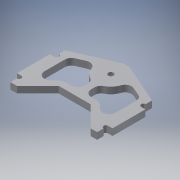
# Autodesk Inventor part: 付け根_サブフレーム_1_3
Saved by Autodesk Inventor 2018 (Build 220112000, 112)
## iProperties
Created: 2016-04-30
Part Number: 付け根_サブフレーム_1_3
Material: アルミニウム 2014-T4
Document SubType Name: Modeling
Designer: hiroaki
Density: 2.8 g/cm^3
Appearance: サテン
Mass: 4.47512 g
Surface Area: 19.2893 cm^2
Volume: 1.59826 cm^3
Author: hiroaki
Autodesk Inventor part; units mm, degrees
ref_plane "YZ Plane" through (0, 0, 0) normal (1, 0, 0) x (0, 1, 0)
ref_plane "XZ Plane" through (0, 0, 0) normal (0, 1, 0) x (-1, 0, 0)
ref_plane "XY Plane" through (0, 0, 0) normal (0, 0, 1) x (1, 0, 0)
sketch "スケッチ1" plane through (0, 0, 0) normal (0, 0, 1) x (1, 0, 0)
  circle A0 centre (0, 0) radius 1.2
  line L0 (-19.75, -6) -> (-21.75, -6)
  line L1 (-21.75, -6) -> (-21.75, -21)
  line L2 (-21.75, -21) -> (-19.75, -21)
  line L3 (-19.75, -3.9) -> (-19.75, -1)
  line L4 (19.75, -1) -> (19.75, -3.9)
  line L5 (-19.75, -23.1) -> (-19.75, -26)
  line L6 (19.75, -26) -> (19.75, -23.1)
  line L7 (19.75, -21) -> (21.75, -21)
  line L8 (21.75, -21) -> (21.75, -6)
  line L9 (21.75, -6) -> (19.75, -6)
  line L10 (0, 0) -> (0, -18.5) construction
  line L11 (-21.75, -13.5) -> (21.75, -13.5) construction
  arc A1 (-19.75, -6) -> (-19.75, -3.9) centre (-19.75, -4.95) ccw
  arc A2 (-19.75, -23.1) -> (-19.75, -21) centre (-19.75, -22.05) ccw
  line L12 (-19.75, -26) -> (-16.75, -26)
  line L13 (-16.75, -26) -> (-7.25, -16.5)
  line L14 (-7.25, -16.5) -> (7.25, -16.5)
  line L15 (7.25, -16.5) -> (16.75, -26)
  line L16 (16.75, -26) -> (19.75, -26)
  arc A3 (19.75, -21) -> (19.75, -23.1) centre (19.75, -22.05) ccw
  arc A4 (19.75, -3.9) -> (19.75, -6) centre (19.75, -4.95) ccw
  circle A5 centre (0, 0) radius 7 construction
  line L17 (1.5877, -2.75) -> (-1.5877, -2.75) construction
  line L18 (-1.5877, -2.75) -> (-3.1754, 0) construction
  line L19 (-3.1754, 0) -> (-1.5877, 2.75) construction
  line L20 (-1.5877, 2.75) -> (1.5877, 2.75) construction
  line L21 (1.5877, 2.75) -> (3.1754, 0) construction
  line L22 (3.1754, 0) -> (1.5877, -2.75) construction
  line L23 (-19.75, -1) -> (-1.4642, 7)
  line L24 (-1.4642, 7) -> (1.4642, 7)
  line L25 (1.4642, 7) -> (19.75, -1)
  circle A6 centre (0, 0) radius 3.1754 construction
  point P0 (0, -13.5)
  dimension "d27" = 2.4
  dimension "d35" = 5
  dimension "d37" = 15
  dimension "d42" = 13.5
  dimension "d43" = 1.05
  dimension "d44" = 39.5
  dimension "d45" = 2
  dimension "d47" = 3
  dimension "d48" = 3
  dimension "d49" = 5.5
  dimension "d71" = 14
  constraints: 52 end point, 8 point on circle, 6 centre point, 6 perpendicular, 6 tangent, 6 vertical alignment, 5 horizontal, 5 symmetric about line, 4 coincident, 3 equal radius, 3 midpoint, 2 collinear, 2 parallel, 2 point on line, 2 vertical, 1 horizontal alignment, 15 other
  measures "d27" diameter of A0
  measures "d35" distance from line of L0 L3.end
  measures "d37" distance of L0.end L1.end
  measures "d42" distance from line of point (0, 0) L11
  measures "d43" radius of A1
  measures "d44" distance between parallel lines of L6 L5
  measures "d45" distance between parallel lines of L3 L1
  measures "d47" distance from line of point (0, -13.5) L14
  measures "d48" distance of L5.end L12.end
  measures "d49" distance between parallel lines of L20 L17
  measures "d71" diameter of A5
extrude "押し出し1" add sketch "スケッチ1" along normal blind 3
sketch "スケッチ2" plane through (0, 0, 3) normal (0, 0, 1) x (1, 0, 0)
  circle A0 centre (0, 0) radius 1.2 projected
  line L0 (-21.75, -6) -> (-21.75, -21) projected
  line L1 (-16.75, -26) -> (-7.25, -16.5) projected
  line L2 (-7.25, -16.5) -> (7.25, -16.5) projected
  line L3 (-1.4642, 7) -> (-19.75, -1) projected
  line L4 (-19.75, -1) -> (-19.75, -3.9) projected
  line L5 (-16.25, -2.7433) -> (-16.25, -21.2574)
  line L6 (-16.25, -21.2574) -> (-8.4926, -13.5)
  line L7 (8.4926, -13.5) -> (16.25, -21.2574)
  line L8 (16.25, -21.2574) -> (16.25, -2.7433)
  line L9 (16.25, -2.7433) -> (6.8662, 1.3621)
  line L10 (-16.25, -2.7433) -> (-6.8662, 1.3621)
  line L11 (-8.4926, -13.5) -> (-1.5, -13.5)
  line L12 (-1.5, -13.5) -> (-1.5, -6.8374)
  arc A1 (-6.8662, 1.3621) -> (-1.5, -6.8374) centre (0, 0) ccw
  line L13 (0, 0) -> (0, -16.5) construction
  line L14 (8.4926, -13.5) -> (1.5, -13.5)
  line L15 (1.5, -13.5) -> (1.5, -6.8374)
  arc A2 (1.5, -6.8374) -> (6.8662, 1.3621) centre (0, 0) ccw
  dimension "d53" = 7
  dimension "d54" = 3.5
  dimension "d55" = 3
  dimension "d56" = 3
  dimension "d57" = 3
  dimension "d58" = 1.5
  constraints: 22 end point, 6 symmetric about line, 4 parallel, 4 point on circle, 2 centre point, 2 coincident, 2 horizontal, 2 perpendicular, 1 midpoint
  measures "d53" radius of A1
  measures "d54" distance between parallel lines of L4 L5
  measures "d55" distance between parallel lines of L3 L10
  measures "d56" distance between parallel lines of L1 L6
  measures "d57" distance between parallel lines of L2 L11
  measures "d58" distance between parallel lines of L13 L12
extrude "押し出し2" cut sketch "スケッチ2" against normal blind 10 contours L10 A1 L12 L11 L6 L5 | L14 L15 A2 L9 L8 L7
fillet "フィレット1" radius 3 12 edges at (-16.25, -21.2574, 1.5) (16.25, -21.2574, 1.5) (8.4926, -13.5, 1.5) (1.5, -13.5, 1.5) (-1.5, -13.5, 1.5) (-1.5, -6.8374, 1.5) (1.5, -6.8374, 1.5) (6.8662, 1.3621, 1.5) (-6.8662, 1.3621, 1.5) (16.25, -2.7433, 1.5) (-16.25, -2.7433, 1.5) (-8.4926, -13.5, 1.5)
sketch "スケッチ3" plane through (0, 0, 0) normal (0, 0, -1) x (-1, 0, 0)
  arc A0 (3.15, -6.2512) -> (6.6615, -2.1504) centre (0, 0) ccw projected
  circle A1 centre (0, 0) radius 1.2 projected
  line L0 (2.75, 1.5877) -> (2.75, -1.5877)
  line L1 (2.75, -1.5877) -> (0, -3.1754)
  line L2 (0, -3.1754) -> (-2.75, -1.5877)
  line L3 (-2.75, -1.5877) -> (-2.75, 1.5877)
  line L4 (-2.75, 1.5877) -> (0, 3.1754)
  line L5 (0, 3.1754) -> (2.75, 1.5877)
  line L6 (2.8, 1.6166) -> (2.8, -1.6166)
  line L7 (2.8, -1.6166) -> (0, -3.2332)
  line L8 (0, -3.2332) -> (-2.8, -1.6166)
  line L9 (-2.8, -1.6166) -> (-2.8, 1.6166)
  line L10 (-2.8, 1.6166) -> (0, 3.2332)
  line L11 (0, 3.2332) -> (2.8, 1.6166)
  circle A2 centre (0, 2.1832) radius 1.05
  circle A3 centre (-1.8907, 1.0916) radius 1.05
  circle A4 centre (-1.8907, -1.0916) radius 1.05
  circle A5 centre (0, -2.1832) radius 1.05
  circle A6 centre (1.8907, -1.0916) radius 1.05
  circle A7 centre (1.8907, 1.0916) radius 1.05
  point P0 (-2.8, 1.6166)
  point P1 (-2.8, -1.6166)
  point P2 (0, -3.2332)
  point P3 (2.8, -1.6166)
  point P4 (2.8, 1.6166)
  dimension "d63" = 2.1
  dimension "d62" = 5.5
  dimension "d64" = 0.05
  dimension "d67" = 360
  constraints: 24 end point, 3 vertical alignment, 1 coincident, 1 vertical, 53 other
  measures "d62" distance between parallel lines of L0 L3
  measures "d64" distance between parallel lines of L11 L5
extrude "押し出し3" cut sketch "スケッチ3" against normal blind 2 contours A1 A7 L0 A6 | A7 A1 | A1 A7 L5 L0 | A6 L0 L1 A1 | A1 A6 | A1 A2 L5 A7 | A7 L6 A6 L0 | L0 L5 A7 L11 L6 | A6 L1 A5 A1 | A6 L6 L7 L1 L0 | A2 A1 | A1 A2 L4 L5 | L5 A2 L11 A7 | L6 A7 | A5 L1 L2 A1 | A1 A5 | A6 L7 A5 L1 | A6 L6 | A1 A3 L4 A2 | L5 L4 A2 L10 L11 | A7 L11 | A5 L2 A4 A1 | A5 L7 L8 L2 L1 | L7 A6 | A3 A1 | A1 A3 L3 L4 | L4 A3 L10 A2 | L11 A2 | A4 L2 L3 A1 | A1 A4 | A5 L8 A4 L2 | A5 L7 | A1 A4 L3 A3 | L4 L3 A3 L9 L10 | A2 L10 | A4 L8 L9 L3 L2 | L8 A5 | L3 A4 L9 A3 | L10 A3 | A4 L8 | A3 L9 | L9 A4
equation "\"d35\" = d3"
equation "\"d37\" = d2"
equation "\"d56\" = d55"
equation "\"d57\" = d56"
equation "\"d58\" = 0.5 * d57"
equation "\"d2\" = 15"
equation "\"d3\" = 5"
equation "\"d8\" = 15"
